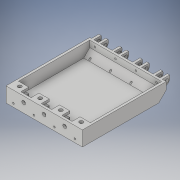
# Autodesk Inventor part: palm
Saved by Autodesk Inventor 2019 (Build 230136000, 136)
## iProperties
Created: 2018-09-20
Part Number: palm
Material: Generic
Document SubType Name: Modeling
Designer: jerem
Density: 1 g/cm^3
Appearance: Default
Author: jerem
Autodesk Inventor part; units mm, degrees
ref_plane "YZ Plane" through (0, 0, 0) normal (1, 0, 0) x (0, 1, 0)
sketch "Sketch1" plane through (0, 0, 0) normal (1, 0, 0) x (0, 1, 0)
  line L0 (-2.6, 0) -> (15.6, 0) projected
  line L1 (0, -98.5723) -> (0, 16.4287) projected
  line L2 (13, 0) -> (0, 0)
  line L3 (13, 0) -> (13, -80)
  line L4 (0, 0) -> (0, -67)
  line L5 (0, -67) -> (6.5, -73.5)
  line L6 (0, -67) -> (9.1924, -67) construction
  arc A0 (6.5, -73.5) -> (13, -80) centre (11.1419, -75.3581) ccw
  circle A1 centre (9.75, -77.5) radius 1.625
  dimension "d2" = 13
  dimension "d6" = 80
  dimension "d7" = 67
  dimension "d8" = 45
  dimension "d9" = 6.5
  dimension "d10" = 5
  dimension "d11" = 3.25
  dimension "d12" = 3.25
  dimension "d13" = 2.5
  constraints: 10 end point, 2 centre point, 2 collinear, 2 horizontal, 2 point on circle, 2 vertical, 1 equal length
  measures "d2" distance of L2.start L2.end
  measures "d6" distance of L2.start L3.end
  measures "d7" distance of L2.end L4.end
  measures "d8" angle of L5 L6
  measures "d9" horizontal distance of L4.end L5.end
  measures "d10" radius of A0
  measures "d11" diameter of A1
  measures "d12" distance from line of L3 A1.centre
  measures "d13" vertical distance of A1.centre L3.end
extrude "Extrusion1" add sketch "Sketch1" along normal mid plane 67
sketch "Sketch3" plane through (-33.5, 13, 0) normal (0, 1, 0) x (1, 0, 0)
  line L0 (0, 73.5) -> (67, 73.5) projected
  line L1 (0, 0) -> (0, 80) projected
  line L2 (67, 80) -> (67, 0) projected
  line L3 (1.5, 73.5) -> (0, 73.5)
  line L4 (0, 73.5) -> (0, 80.5)
  line L5 (0, 80.5) -> (1.5, 80.5)
  line L6 (1.5, 80.5) -> (1.5, 73.5)
  line L7 (7.5, 73.5) -> (3.5, 73.5)
  line L8 (3.5, 73.5) -> (3.5, 80.5)
  line L9 (3.5, 80.5) -> (7.5, 80.5)
  line L10 (7.5, 80.5) -> (7.5, 73.5)
  line L11 (19.5, 73.5) -> (9.5, 73.5)
  line L12 (9.5, 73.5) -> (9.5, 80.5)
  line L13 (9.5, 80.5) -> (19.5, 80.5)
  line L14 (19.5, 80.5) -> (19.5, 73.5)
  line L15 (25.5, 80.5) -> (21.5, 80.5)
  line L16 (21.5, 80.5) -> (21.5, 73.5)
  line L17 (21.5, 73.5) -> (25.5, 73.5)
  line L18 (25.5, 73.5) -> (25.5, 80.5)
  line L19 (37.5, 73.5) -> (27.5, 73.5)
  line L20 (27.5, 73.5) -> (27.5, 80.5)
  line L21 (27.5, 80.5) -> (37.5, 80.5)
  line L22 (37.5, 80.5) -> (37.5, 73.5)
  line L23 (43.5, 73.5) -> (39.5, 73.5)
  line L24 (39.5, 73.5) -> (39.5, 80.5)
  line L25 (39.5, 80.5) -> (43.5, 80.5)
  line L26 (43.5, 80.5) -> (43.5, 73.5)
  line L27 (55.5, 73.5) -> (45.5, 73.5)
  line L28 (45.5, 73.5) -> (45.5, 80.5)
  line L29 (45.5, 80.5) -> (55.5, 80.5)
  line L30 (55.5, 80.5) -> (55.5, 73.5)
  line L31 (61.5, 73.5) -> (57.5, 73.5)
  line L32 (57.5, 73.5) -> (57.5, 80.5)
  line L33 (57.5, 80.5) -> (61.5, 80.5)
  line L34 (61.5, 80.5) -> (61.5, 73.5)
  line L35 (67, 73.5) -> (63.5, 73.5)
  line L36 (63.5, 73.5) -> (63.5, 80.5)
  line L37 (63.5, 80.5) -> (67, 80.5)
  line L38 (67, 80.5) -> (67, 73.5)
  point P0 (33.5, 0)
  dimension "d52" = 1.5
  dimension "d53" = 7
  dimension "d54" = 4
  dimension "d55" = 7
  dimension "d56" = 2
  dimension "d57" = 10
  dimension "d58" = 7
  dimension "d59" = 2
  dimension "d60" = 4
  dimension "d61" = 7
  dimension "d62" = 2
  dimension "d63" = 10
  dimension "d64" = 7
  dimension "d65" = 2
  dimension "d66" = 4
  dimension "d67" = 2
  dimension "d68" = 7
  dimension "d69" = 10
  dimension "d70" = 7
  dimension "d71" = 2
  dimension "d72" = 4
  dimension "d73" = 7
  dimension "d74" = 2
  dimension "d75" = 7
  dimension "d76" = 2
  constraints: 72 end point, 18 parallel, 11 collinear, 9 horizontal, 9 perpendicular
  measures "d52" distance of L4.end L5.end
  measures "d53" distance of L3.end L4.end
  measures "d54" distance of L8.end L9.end
  measures "d55" distance of L7.end L8.end
  measures "d56" distance between parallel lines of L6 L8
  measures "d57" distance of L12.end L13.end
  measures "d58" distance of L11.end L12.end
  measures "d59" distance between parallel lines of L10 L12
  measures "d60" distance of L17.end L16.end
  measures "d61" distance of L16.end L15.end
  measures "d62" distance between parallel lines of L16 L14
  measures "d63" distance of L20.end L22.start
  measures "d64" distance of L20.start L20.end
  measures "d65" distance between parallel lines of L18 L20
  measures "d66" distance of L24.end L25.end
  measures "d67" distance between parallel lines of L22 L24
  measures "d68" distance between parallel lines of L0 L25
  measures "d69" distance of L28.end L30.start
  measures "d70" distance of L28.start L28.end
  measures "d71" distance between parallel lines of L26 L28
  measures "d72" distance of L32.end L33.end
  measures "d73" distance of L31.end L32.end
  measures "d74" distance between parallel lines of L32 L30
  measures "d75" distance of L35.end L36.end
  measures "d76" distance between parallel lines of L34 L36
extrude "Extrusion3" cut sketch "Sketch3" against normal blind 13
ref_plane "Work Plane1" through (31.5, 0, 0) normal (1, 0, 0) x (0, 0, -1)
sketch "Sketch4" plane through (31.5, 0, 0) normal (1, 0, 0) x (0, 0, -1)
  line L0 (2, 13) -> (2, 2)
  line L1 (2, 2) -> (66.1716, 2)
  line L2 (0, 13) -> (73.5, 13) projected
  line L3 (0, 0) -> (0, 13) projected
  line L4 (67, 0) -> (0, 0) projected
  line L5 (73.5, 6.5) -> (67, 0) projected
  line L6 (71.5, 7.3284) -> (71.5, 13)
  line L7 (73.5, 13) -> (73.5, 6.5) projected
  line L8 (71.5, 7.3284) -> (66.1716, 2)
  dimension "d80" = 2
  dimension "d81" = 2
  dimension "d82" = 2
  dimension "d83" = 2
  dimension "d84" = 2
  constraints: 8 end point, 2 perpendicular, 2 point on line, 1 vertical
  measures "d80" distance between parallel lines of L0 L3
  measures "d81" distance between parallel lines of L4 L1
  measures "d82" distance from line of L5 L1.end
  measures "d83" distance between parallel lines of L7 L6
  measures "d84" distance from line of L5 L6.start
extrude "Extrusion4" cut sketch "Sketch4" against normal blind 63 contours L2 L6 L8 L1 L0
sketch "Sketch5" plane through (4, 13, -73.5) normal (0, 0, -1) x (-1, 0, 0)
  line L0 (4, -15.6) -> (4, 2.6) projected
  line L1 (50.9, -13) -> (-42.9, -13) projected
  line L2 (-29.5, -6.5) -> (-29.5, 0) projected
  line L3 (37.5, 0) -> (37.5, -6.5) projected
  line L4 (-18, 0) -> (-8, 0) projected
  circle A0 centre (-23, -3) radius 0.75
  circle A1 centre (-5, -3) radius 0.75
  circle A2 centre (13, -3) radius 0.75
  line L5 (0, 0) -> (10, 0) projected
  circle A3 centre (31, -3) radius 0.75
  dimension "d88" = 1.5
  dimension "d89" = 3
  dimension "d90" = 6.5
  dimension "d94" = 1.5
  dimension "d95" = 3
  dimension "d96" = 18
  dimension "d100" = 1.5
  dimension "d101" = 3
  dimension "d102" = 18
  dimension "d106" = 1.5
  dimension "d108" = 3
  dimension "d109" = 18
  constraints: 4 centre point
  measures "d88" diameter of A0
  measures "d89" distance from line of L4 A0.centre
  measures "d90" distance from line of L2 A0.centre
  measures "d94" diameter of A1
  measures "d95" distance from line of L4 A1.centre
  measures "d96" distance of A0.centre A1.centre
  measures "d100" diameter of A2
  measures "d101" distance from line of L5 A2.centre
  measures "d102" distance of A2.centre A1.centre
  measures "d106" diameter of A3
  measures "d108" distance from line of A3.centre L5
  measures "d109" distance of A3.centre A2.centre
ref_plane "Work Plane2" through (-33.5, 0, -33.5) normal (0, 0, 1) x (1, 0, 0)
extrude "Extrusion11" cut sketch "Sketch5" against normal blind 2
sketch "Sketch13" plane through (22, 13, -73.5) normal (0, 0, -1) x (-1, 0, 0)
  line L0 (55.5, -13) -> (-11.5, -13) projected
  circle A0 centre (-5, -10) radius 0.75
  circle A1 centre (13, -10) radius 0.75
  circle A2 centre (31, -10) radius 0.75
  circle A3 centre (49, -10) radius 0.75
  line L1 (-11.5, -13) -> (-11.5, -6.5) projected
  line L2 (55.5, -6.5) -> (55.5, -13) projected
  point P0 (22, -13)
  dimension "d159" = 1.5
  dimension "d160" = 1.5
  dimension "d161" = 1.5
  dimension "d162" = 1.5
  dimension "d163" = 3
  dimension "d164" = 6.5
  dimension "d165" = 3
  dimension "d166" = 18
  dimension "d167" = 3
  dimension "d168" = 18
  dimension "d169" = 3
  dimension "d170" = 18
  constraints: 4 centre point
  measures "d159" diameter of A0
  measures "d160" diameter of A1
  measures "d161" diameter of A2
  measures "d162" diameter of A3
  measures "d163" distance from line of L0 A0.centre
  measures "d164" distance from line of L1 A0.centre
  measures "d165" distance from line of L0 A1.centre
  measures "d166" distance of A0.centre A1.centre
  measures "d167" distance from line of L0 A2.centre
  measures "d168" distance of A2.centre A1.centre
  measures "d169" distance from line of L0 A3.centre
  measures "d170" distance of A3.centre A2.centre
extrude "Extrusion12" cut sketch "Sketch13" against normal through all
sketch "Sketch22" plane through (-33.5, 13, 0) normal (0, 1, 0) x (1, 0, 0)
  line L0 (65, 2) -> (2, 2) projected
  line L1 (2, 9) -> (11, 9)
  line L2 (11, 9) -> (11, 2)
  line L3 (11, 2) -> (2, 2)
  line L4 (2, 2) -> (2, 9)
  circle A0 centre (6.5, 67.1716) radius 0.75 projected
  line L5 (65, 2) -> (65, 66.1716) projected
  line L6 (65, 66.1716) -> (2, 66.1716) projected
  line L7 (2, 66.1716) -> (2, 2) projected
  line L8 (65, 2) -> (2, 2) projected
  line L9 (20, 9) -> (29, 9)
  line L10 (29, 9) -> (29, 2)
  line L11 (29, 2) -> (20, 2)
  line L12 (20, 2) -> (20, 9)
  line L13 (56, 9) -> (65, 9)
  line L14 (65, 9) -> (65, 2)
  line L15 (65, 2) -> (56, 2)
  line L16 (56, 2) -> (56, 9)
  line L17 (38, 9) -> (47, 9)
  line L18 (47, 9) -> (47, 2)
  line L19 (47, 2) -> (38, 2)
  line L20 (38, 2) -> (38, 9)
  dimension "d275" = 9
  dimension "d278" = 7
  dimension "d279" = 9
  dimension "d280" = 7
  dimension "d281" = 9
  dimension "d282" = 9
  dimension "d283" = 7
  dimension "d284" = 9
  dimension "d285" = 7
  dimension "d286" = 9
  constraints: 32 end point, 8 parallel, 6 collinear, 4 horizontal, 4 perpendicular
  measures "d275" distance of L2.end L3.end
  measures "d278" distance between parallel lines of L0 L1
  measures "d279" distance of L10.end L11.end
  measures "d280" distance of L9.end L10.end
  measures "d281" distance between parallel lines of L12 L2
  measures "d282" distance of L14.end L15.end
  measures "d283" distance of L13.end L14.end
  measures "d284" distance of L18.end L19.end
  measures "d285" distance of L17.end L18.end
  measures "d286" distance between parallel lines of L16 L18
extrude "Extrusion19" add sketch "Sketch22" against normal blind 7 contours L0 L16 L13 L5 | L0 L20 L17 L18 | L0 L12 L9 L10 | L1 L2 L0 L4
sketch "Sketch23" plane through (31.5, 0, 0) normal (-1, 0, 0) x (0, 0, 1)
  line L0 (-9.5, 11) -> (-2, 11)
  line L1 (-2, 11) -> (-2, 8)
  line L2 (-2, 8) -> (-9.5, 8)
  line L3 (-9.5, 8) -> (-9.5, 11)
  line L4 (-2, 13) -> (-2, 6) projected
  line L5 (-2, 13) -> (-9, 13) projected
  point P0 (0, 0)
  dimension "d289" = 7.5
  dimension "d290" = 3
  dimension "d291" = 2
  constraints: 8 end point, 2 parallel, 1 collinear, 1 horizontal, 1 perpendicular
  measures "d289" distance of L1.end L2.end
  measures "d290" distance of L0.end L1.end
  measures "d291" distance between parallel lines of L5 L0
extrude "Extrusion20" cut sketch "Sketch23" along normal blind 63
sketch "Sketch24" plane through (-33.5, 13, 0) normal (0, 1, 0) x (1, 0, 0)
  line L0 (56, 9) -> (65, 9) projected
  line L1 (56, 2) -> (56, 9) projected
  line L2 (47, 9) -> (47, 2) projected
  line L3 (38, 9) -> (47, 9) projected
  line L4 (29, 9) -> (29, 2) projected
  line L5 (20, 9) -> (29, 9) projected
  line L6 (11, 9) -> (11, 2) projected
  line L7 (2, 9) -> (11, 9) projected
  circle A0 centre (60.5, 5.5) radius 1.625
  circle A1 centre (42.5, 5.5) radius 1.625
  circle A2 centre (24.5, 5.5) radius 1.625
  circle A3 centre (6.5, 5.5) radius 1.625
  point P0 (33.5, 0)
  dimension "d294" = 3.25
  dimension "d295" = 3.5
  dimension "d296" = 4.5
  dimension "d297" = 3.25
  dimension "d298" = 3.5
  dimension "d299" = 4.5
  dimension "d301" = 3.25
  dimension "d302" = 3.5
  dimension "d303" = 4.5
  dimension "d304" = 3.25
  dimension "d305" = 3.5
  dimension "d306" = 4.5
  constraints: 4 centre point
  measures "d294" diameter of A0
  measures "d295" distance from line of L0 A0.centre
  measures "d296" distance from line of L1 A0.centre
  measures "d297" diameter of A1
  measures "d298" distance from line of L3 A1.centre
  measures "d299" distance from line of L2 A1.centre
  measures "d301" diameter of A2
  measures "d302" distance from line of L5 A2.centre
  measures "d303" distance from line of L4 A2.centre
  measures "d304" diameter of A3
  measures "d305" distance from line of L7 A3.centre
  measures "d306" distance from line of L6 A3.centre
extrude "Extrusion21" cut sketch "Sketch24" against normal blind 7
sketch "Sketch26" plane through (31.5, 2, -2) normal (0, 0, -1) x (-1, 0, 0)
  line L0 (9, 6) -> (9, 4) projected
  line L1 (9, 11) -> (9, 9) projected
  line L2 (0, 6) -> (9, 6) projected
  line L3 (0, 9) -> (9, 9) projected
  line L4 (0, 9) -> (9, 9) projected
  line L5 (18, 9) -> (18, 11) projected
  line L6 (18, 6) -> (27, 6) projected
  line L7 (36, 6) -> (45, 6) projected
  line L8 (54, 6) -> (63, 6) projected
  circle A0 centre (13.5, 6) radius 1.625
  circle A1 centre (31.5, 6) radius 1.625
  circle A2 centre (49.5, 6) radius 1.625
  point P0 (31.5, -2)
  dimension "d311" = 3.25
  dimension "d313" = 4.5
  dimension "d314" = 3.25
  dimension "d316" = 4.5
  dimension "d317" = 3.25
  dimension "d319" = 4.5
  constraints: 3 centre point, 3 point on line
  measures "d311" diameter of A0
  measures "d313" distance from line of L0 A0.centre
  measures "d314" diameter of A1
  measures "d316" distance of L6.end A1.centre
  measures "d317" diameter of A2
  measures "d319" distance of A2.centre L7.end
extrude "Extrusion22" cut sketch "Sketch26" against normal blind 2
body "Solid1"
